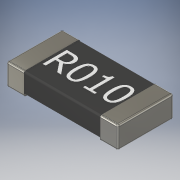
# Autodesk Inventor part: Resistor_1608-0.5mm
Saved by Autodesk Inventor 2018 (Build 220112000, 112)
## iProperties
Created: 2016-08-15
Part Number: Resistor_1608-0.5mm
Material: Copper
Document SubType Name: Modeling
Designer: Bradley
Density: 8.94 g/cm^3
Appearance: Smooth - Black
Author: Bradley
Autodesk Inventor part; units mm, degrees
ref_plane "YZ Plane" through (0, 0, 0) normal (1, 0, 0) x (0, 1, 0)
ref_plane "XZ Plane" through (0, 0, 0) normal (0, 1, 0) x (-1, 0, 0)
ref_plane "XY Plane" through (0, 0, 0) normal (0, 0, 1) x (1, 0, 0)
sketch "Sketch1" plane through (0, 0, 0) normal (0, 0, 1) x (1, 0, 0)
  line L0 (-1.6, 0.585) -> (-1.092, 0.585)
  line L1 (-1.092, 0.585) -> (-1.092, -0.05)
  line L2 (-1.092, -0.05) -> (-1.6, -0.05)
  line L3 (-1.6, -0.05) -> (-1.6, 0.585)
  line L4 (-1.092, 0.575) -> (1.092, 0.575)
  line L5 (1.092, 0.575) -> (1.092, 0)
  line L6 (1.092, 0) -> (-1.092, 0)
  line L7 (-1.092, 0) -> (-1.092, 0.575)
  line L8 (1.092, 0.585) -> (1.6, 0.585)
  line L9 (1.6, 0.585) -> (1.6, -0.05)
  line L10 (1.6, -0.05) -> (1.092, -0.05)
  line L11 (1.092, -0.05) -> (1.092, 0.585)
  point P0 (0, 0)
  point P1 (0, 0.575)
  point P2 (0, 0)
  dimension "d0" = 3.2
  dimension "d1" = 0.635
  dimension "d2" = 0.508
  dimension "d3" = 0.05
  dimension "d6" = 0.01
  constraints: 24 end point, 6 parallel, 3 horizontal, 3 perpendicular, 3 point on line, 2 collinear, 2 midpoint, 1 coincident, 1 vertical alignment
  measures "d0" distance between parallel lines of L9 L3
  measures "d1" distance of L2.end L0.start
  measures "d2" distance of L1.end L2.end
  measures "d3" distance between parallel lines of L2 L6
  measures "d6" distance between parallel lines of L4 L0
extrude "Extrusion1" add sketch "Sketch1" along normal mid plane 1.6 contours L0 L1 L2 L3 | L11 L8 L9 L10 L5
extrude "Extrusion2" add sketch "Sketch1" along normal mid plane 1.59 contours L4 L5 L6 L1
sketch "Sketch3" plane through (-1.092, 0.575, 0.84) normal (0, 1, 0) x (1, 0, 0)
  line L0 (0, 0.045) -> (0, 1.635) projected
  line L1 (2.184, 0.045) -> (0, 0.045) projected
  line L2 (2.184, 1.635) -> (2.184, 0.045) projected
  line L3 (0, 1.635) -> (2.184, 1.635) projected
  line L4 (2.184, 1.64) -> (2.184, 0.04) construction
  line L5 (2.184, 0.84) -> (0, 0.84) construction
  line L6 (0, 1.64) -> (0, 0.04) construction
  line L7 (0.6181, 0.49) -> (0.4972, 0.49)
  line L8 (0.4972, 0.49) -> (0.276, 0.7685)
  line L9 (0.276, 0.7685) -> (0.1694, 0.7685)
  line L10 (0.1694, 0.7685) -> (0.1694, 0.49)
  line L11 (0.1694, 0.49) -> (0.0763, 0.49)
  line L12 (0.0763, 0.49) -> (0.0763, 1.19)
  line L13 (0.0763, 1.19) -> (0.2567, 1.19)
  spline S0 degree 2 poles (0.2567, 1.19) (0.3168, 1.19) (0.398, 1.177) (0.4348, 1.1531) knots 0 0 0 1 2 2 2
  spline S1 degree 2 poles (0.4348, 1.1531) (0.4717, 1.1293) (0.5142, 1.055) (0.5142, 1) knots 0 0 0 1 2 2 2
  spline S2 degree 2 poles (0.5142, 1) (0.5142, 0.9234) (0.436, 0.8196) (0.369, 0.7946) knots 0 0 0 1 2 2 2
  line L14 (0.369, 0.7946) -> (0.6181, 0.49)
  spline S3 degree 2 poles (0.4172, 0.9926) (0.4172, 1.0232) (0.3957, 1.0703) (0.373, 1.0856) knots 0 0 0 1 2 2 2
  spline S4 degree 2 poles (0.373, 1.0856) (0.3531, 1.0987) (0.3004, 1.1094) (0.2618, 1.1094) knots 0 0 0 1 2 2 2
  line L15 (0.2618, 1.1094) -> (0.1694, 1.1094)
  line L16 (0.1694, 1.1094) -> (0.1694, 0.8462)
  line L17 (0.1694, 0.8462) -> (0.251, 0.8462)
  spline S5 degree 2 poles (0.251, 0.8462) (0.2913, 0.8462) (0.3554, 0.8604) (0.3775, 0.8825) knots 0 0 0 1 2 2 2
  spline S6 degree 2 poles (0.3775, 0.8825) (0.398, 0.9018) (0.4172, 0.9563) (0.4172, 0.9926) knots 0 0 0 1 2 2 2
  spline S7 degree 2 poles (1.0894, 0.84) (1.0894, 0.6517) (0.98, 0.4753) (0.8659, 0.4753) knots 0 0 0 1 2 2 2
  spline S8 degree 2 poles (0.8659, 0.4753) (0.7502, 0.4753) (0.6419, 0.6551) (0.6419, 0.8394) knots 0 0 0 1 2 2 2
  spline S9 degree 2 poles (0.6419, 0.8394) (0.6419, 1.0289) (0.7514, 1.2042) (0.8659, 1.2042) knots 0 0 0 1 2 2 2
  spline S10 degree 2 poles (0.8659, 1.2042) (0.9811, 1.2042) (1.0894, 1.0227) (1.0894, 0.84) knots 0 0 0 1 2 2 2
  spline S11 degree 2 poles (0.9692, 0.6267) (0.9828, 0.6613) (0.9941, 0.768) (0.9941, 0.84) knots 0 0 0 1 2 2 2
  spline S12 degree 2 poles (0.9941, 0.84) (0.9941, 0.912) (0.9828, 1.0181) (0.9686, 1.0539) knots 0 0 0 1 2 2 2
  spline S13 degree 2 poles (0.9686, 1.0539) (0.9544, 1.0896) (0.9051, 1.1265) (0.8659, 1.1265) knots 0 0 0 1 2 2 2
  spline S14 degree 2 poles (0.8659, 1.1265) (0.8268, 1.1265) (0.7763, 1.0896) (0.7616, 1.0527) knots 0 0 0 1 2 2 2
  spline S15 degree 2 poles (0.7616, 1.0527) (0.7474, 1.017) (0.7372, 0.9081) (0.7372, 0.8394) knots 0 0 0 1 2 2 2
  spline S16 degree 2 poles (0.7372, 0.8394) (0.7372, 0.7657) (0.7463, 0.667) (0.761, 0.6284) knots 0 0 0 1 2 2 2
  spline S17 degree 2 poles (0.761, 0.6284) (0.7746, 0.5921) (0.8251, 0.553) (0.8659, 0.553) knots 0 0 0 1 2 2 2
  spline S18 degree 2 poles (0.8659, 0.553) (0.9045, 0.553) (0.955, 0.5898) (0.9692, 0.6267) knots 0 0 0 1 2 2 2
  line L18 (1.5756, 0.49) -> (1.2341, 0.49)
  line L19 (1.2341, 0.49) -> (1.2341, 0.5615)
  line L20 (1.2341, 0.5615) -> (1.3612, 0.5615)
  line L21 (1.3612, 0.5615) -> (1.3612, 1.0306)
  line L22 (1.3612, 1.0306) -> (1.2341, 1.0306)
  line L23 (1.2341, 1.0306) -> (1.2341, 1.0947)
  spline S19 degree 2 poles (1.2341, 1.0947) (1.3061, 1.0947) (1.3742, 1.1355) (1.3788, 1.1923) knots 0 0 0 1 2 2 2
  line L24 (1.3788, 1.1923) -> (1.4514, 1.1923)
  line L25 (1.4514, 1.1923) -> (1.4514, 0.5615)
  line L26 (1.4514, 0.5615) -> (1.5756, 0.5615)
  line L27 (1.5756, 0.5615) -> (1.5756, 0.49)
  spline S20 degree 2 poles (2.14, 0.84) (2.14, 0.6517) (2.0305, 0.4753) (1.9165, 0.4753) knots 0 0 0 1 2 2 2
  spline S21 degree 2 poles (1.9165, 0.4753) (1.8008, 0.4753) (1.6924, 0.6551) (1.6924, 0.8394) knots 0 0 0 1 2 2 2
  spline S22 degree 2 poles (1.6924, 0.8394) (1.6924, 1.0289) (1.8019, 1.2042) (1.9165, 1.2042) knots 0 0 0 1 2 2 2
  spline S23 degree 2 poles (1.9165, 1.2042) (2.0317, 1.2042) (2.14, 1.0227) (2.14, 0.84) knots 0 0 0 1 2 2 2
  spline S24 degree 2 poles (2.0198, 0.6267) (2.0334, 0.6613) (2.0447, 0.768) (2.0447, 0.84) knots 0 0 0 1 2 2 2
  spline S25 degree 2 poles (2.0447, 0.84) (2.0447, 0.912) (2.0334, 1.0181) (2.0192, 1.0539) knots 0 0 0 1 2 2 2
  spline S26 degree 2 poles (2.0192, 1.0539) (2.005, 1.0896) (1.9557, 1.1265) (1.9165, 1.1265) knots 0 0 0 1 2 2 2
  spline S27 degree 2 poles (1.9165, 1.1265) (1.8774, 1.1265) (1.8269, 1.0896) (1.8121, 1.0527) knots 0 0 0 1 2 2 2
  spline S28 degree 2 poles (1.8121, 1.0527) (1.798, 1.017) (1.7877, 0.9081) (1.7877, 0.8394) knots 0 0 0 1 2 2 2
  spline S29 degree 2 poles (1.7877, 0.8394) (1.7877, 0.7657) (1.7968, 0.667) (1.8116, 0.6284) knots 0 0 0 1 2 2 2
  spline S30 degree 2 poles (1.8116, 0.6284) (1.8252, 0.5921) (1.8757, 0.553) (1.9165, 0.553) knots 0 0 0 1 2 2 2
  spline S31 degree 2 poles (1.9165, 0.553) (1.9551, 0.553) (2.0056, 0.5898) (2.0198, 0.6267) knots 0 0 0 1 2 2 2
  point P0 (1.092, 0.84)
  point P1 (1.092, 0.84)
  constraints: 4 midpoint, 2 end point, 1 horizontal, 1 perpendicular
extrude "Extrusion4" add sketch "Sketch3" along normal blind 0.01 contours L7 L8 L9 L10 L11 L12 L13 S0 S1 S2 L14 | S7 S8 S9 S10 | L18 L19 L20 L21 L22 L23 S19 L24 L25 L26 L27 | S20 S21 S22 S23
fillet "Fillet2" radius 0.05 4 edges at (0, 0.575, 0.795) (0, 0, 0.795) (0, 0.575, -0.795) (0, 0, -0.795)
fillet "Fillet1" radius 0.05 16 edges at (-1.346, 0.585, 0.8) (1.346, 0.585, 0.8) (-1.346, 0.585, -0.8) (1.346, 0.585, -0.8) (1.6, 0.585, 0) (1.6, 0.2675, -0.8) (1.6, -0.05, 0) (1.346, -0.05, -0.8) (1.346, -0.05, 0.8) (1.6, 0.2675, 0.8) (-1.346, -0.05, -0.8) (-1.6, -0.05, 0) (-1.6, 0.2675, 0.8) (-1.346, -0.05, 0.8) (-1.6, 0.2675, -0.8) (-1.6, 0.585, 0)
body "Solid1"
